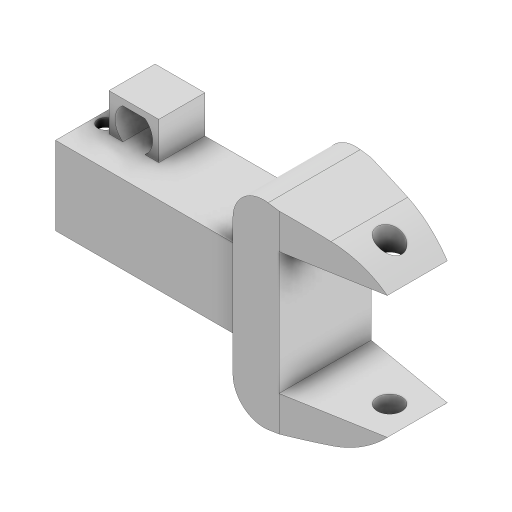
# Autodesk Inventor part: Nuckle
Saved by Autodesk Inventor 2023 (Build 270158000, 158)
## iProperties
Created: 2023-03-23
Part Number: Nuckle
Material: Generic
Document SubType Name: Modeling
Designer: Juyoung Han
Density: 1 g/cm^3
Appearance: Default
Author: Juyoung Han
Autodesk Inventor part; units mm, degrees
ref_plane "YZ Plane" through (0, 0, 0) normal (1, 0, 0) x (0, 1, 0)
ref_plane "XZ Plane" through (0, 0, 0) normal (0, 1, 0) x (-1, 0, 0)
ref_plane "XY Plane" through (0, 0, 0) normal (0, 0, 1) x (1, 0, 0)
sketch "Sketch1" plane through (0, 0, 0) normal (0, 0, 1) x (1, 0, 0)
  line L0 (0, 20) -> (30, 20)
  line L1 (0, 20) -> (0, 0)
  line L2 (-45, 20) -> (-45, 35)
  arc A0 (30, 25) -> (-45, 35) centre (-45, -251.25) ccw
  line L3 (-45, 20) -> (-45, 0)
  line L4 (0, -20) -> (30, -20)
  line L5 (45, -20) -> (45, -20.4834)
  line L6 (0, -20) -> (0, 0)
  line L7 (-45, -20) -> (-45, -35)
  arc A1 (-45, -35) -> (30, -25) centre (-45, 251.25) ccw
  line L8 (-45, -20) -> (-45, 0)
  line L9 (30, 25) -> (30, 20)
  line L10 (30, -25) -> (30, -20)
  point P0 (45, 20.4834)
  point P1 (45, 22.5)
  point P2 (30, 37.5)
  point P3 (-25, -20)
  point P4 (0, -32.987)
  point P5 (45, -22.5)
  point P6 (30, -37.5)
  point P7 (45, -22.5)
  point P8 (30, -37.5)
  dimension "d17" = 15
  constraints: 22 end point, 6 point on circle, 3 point on line, 2 centre point, 2 vertical, 1 horizontal, 1 perpendicular
  measures "d17" distance of L2.start L2.end
extrude "Extrusion1" add sketch "Sketch1" along normal mid plane 30
sketch "Sketch3" plane through (0, -20, 15) normal (0, 1, 0) x (1, 0, 0)
  line L0 (0, 0) -> (0, 30) projected
  line L1 (30, 0) -> (0, 0) projected
  line L2 (0, 30) -> (30, 30) projected
  circle A0 centre (36.5, 15) radius 2
  line L3 (30, 30) -> (30, 0) projected
  point P0 (0, 15)
  dimension "d18" = 4
  constraints: 1 centre point
  measures "d18" diameter of A0
extrude "Extrusion3" cut sketch "Sketch3" along normal through all both and the other way through all contours A0
fillet "Fillet3" radius 30 1 edges at (30, 25, 0)
fillet "Fillet4" radius 30 1 edges at (30, -25, 0)
sketch "Sketch6" plane through (-45, -35, 15) normal (-1, 0, 0) x (0, 0, 1)
  line L0 (-24.0585, 25.4415) -> (-25, 24.5) construction
  line L1 (-4.3571, 37.8214) -> (-10.3571, 37.8214)
  line L2 (-10.3571, 37.8214) -> (-10.3571, 31.8214)
  line L3 (-10.3571, 31.8214) -> (-4.5, 31.8214)
  line L4 (-25, 37.8214) -> (-19, 37.8214)
  line L5 (-19, 37.8214) -> (-19, 31.8214)
  line L6 (-19, 31.8214) -> (-25, 31.8214)
  line L7 (-25, 24.5) -> (-25, 31.8214)
  line L8 (-25, 37.8214) -> (-25, 45)
  line L9 (-4.3571, 45) -> (-4.3571, 37.8214)
  line L10 (-4.5, 31.8214) -> (-4.5, 24.5)
  line L11 (-11.6786, 45) -> (-11.6786, 39)
  line L12 (-11.6786, 39) -> (-17.6786, 39)
  line L13 (-17.6786, 39) -> (-17.6786, 45)
  line L14 (-25, 45) -> (-17.6786, 45)
  line L15 (-11.6786, 45) -> (-4.3571, 45)
  line L16 (-17.6786, 24.5) -> (-17.6786, 30.5)
  line L17 (-17.6786, 30.5) -> (-11.6786, 30.5)
  line L18 (-11.6786, 30.5) -> (-11.6786, 24.5)
  line L19 (-4.5, 24.5) -> (-11.6786, 24.5)
  line L20 (-17.6786, 24.5) -> (-25, 24.5)
  dimension "d59" = 20.5
  dimension "d67" = 6
  dimension "d68" = 6
  dimension "d69" = 6
  dimension "d70" = 6
  dimension "d71" = 6
  dimension "d73" = 6
  constraints: 42 end point, 13 perpendicular, 10 parallel, 3 horizontal
  measures "d59" distance of L10.end L0.end
  measures "d67" distance of L1.end L2.end
  measures "d68" distance of L1.start L1.end
  measures "d69" distance of L4.start L4.end
  measures "d70" distance of L4.end L5.end
  measures "d71" distance of L11.end L12.end
  measures "d73" distance of L16.start L16.end
extrude "Extrusion5" cut sketch "Sketch6" against normal blind 42
sketch "Sketch7" plane through (-45, -35, 15) normal (-1, 0, 0) x (0, 0, 1)
  line L0 (-30, 50) -> (0, 50)
  line L1 (0, 50) -> (0, 20)
  line L2 (0, 20) -> (-30, 20)
  line L3 (-30, 20) -> (-30, 50)
  line L4 (-30, 50) -> (0, 20) construction
  line L5 (0, 50) -> (-30, 20) construction
  line L6 (-22.5355, 32.4645) -> (-22.5355, 28.5251) projected
  line L7 (-24.5355, 32.4645) -> (-22.5355, 32.4645) projected
  line L8 (-24.5355, 25.4645) -> (-24.5355, 32.4645) projected
  line L9 (-17.5355, 25.4645) -> (-24.5355, 25.4645) projected
  line L10 (-17.5355, 27.4645) -> (-17.5355, 25.4645) projected
  line L11 (-21.4749, 27.4645) -> (-17.5355, 27.4645) projected
  line L12 (-17.9393, 31) -> (-21.4749, 27.4645) projected
  line L13 (-12.0607, 31) -> (-17.9393, 31) projected
  line L14 (-8.5251, 27.4645) -> (-12.0607, 31) projected
  line L15 (-12.4645, 27.4645) -> (-8.5251, 27.4645) projected
  line L16 (-12.4645, 25.4645) -> (-12.4645, 27.4645) projected
  line L17 (-5.4645, 25.4645) -> (-12.4645, 25.4645) projected
  line L18 (-5.4645, 32.4645) -> (-5.4645, 25.4645) projected
  line L19 (-7.4645, 32.4645) -> (-5.4645, 32.4645) projected
  line L20 (-7.4645, 28.5251) -> (-7.4645, 32.4645) projected
  line L21 (-11, 32.0607) -> (-7.4645, 28.5251) projected
  line L22 (-11, 37.9393) -> (-11, 32.0607) projected
  line L23 (-7.4645, 41.4749) -> (-11, 37.9393) projected
  line L24 (-7.4645, 37.5355) -> (-7.4645, 41.4749) projected
  line L25 (-5.4645, 37.5355) -> (-7.4645, 37.5355) projected
  line L26 (-5.4645, 44.5355) -> (-5.4645, 37.5355) projected
  line L27 (-12.4645, 44.5355) -> (-5.4645, 44.5355) projected
  line L28 (-12.4645, 42.5355) -> (-12.4645, 44.5355) projected
  line L29 (-8.5251, 42.5355) -> (-12.4645, 42.5355) projected
  line L30 (-12.0607, 39) -> (-8.5251, 42.5355) projected
  line L31 (-17.9393, 39) -> (-12.0607, 39) projected
  line L32 (-21.4749, 42.5355) -> (-17.9393, 39) projected
  line L33 (-17.5355, 42.5355) -> (-21.4749, 42.5355) projected
  line L34 (-17.5355, 44.5355) -> (-17.5355, 42.5355) projected
  line L35 (-24.5355, 44.5355) -> (-17.5355, 44.5355) projected
  line L36 (-24.5355, 37.5355) -> (-24.5355, 44.5355) projected
  line L37 (-22.5355, 37.5355) -> (-24.5355, 37.5355) projected
  line L38 (-22.5355, 41.4749) -> (-22.5355, 37.5355) projected
  line L39 (-19, 37.9393) -> (-22.5355, 41.4749) projected
  line L40 (-19, 32.0607) -> (-19, 37.9393) projected
  line L41 (-22.5355, 28.5251) -> (-19, 32.0607) projected
  line L42 (-30, 70) -> (0, 70) projected
  line L43 (-30, 0) -> (-30, 70) projected
  line L44 (0, 70) -> (0, 0) projected
  line L45 (-30, 0) -> (0, 0) projected
  point P0 (-15, 35)
  dimension "d47" = 30
  dimension "d48" = 30
  constraints: 12 end point, 2 midpoint, 2 parallel, 1 horizontal, 1 perpendicular
  measures "d47" distance of L1.end L2.end
  measures "d48" distance of L0.end L1.end
extrude "Extrusion6" cut sketch "Sketch7" against normal blind 30 contours L43 L42 L44 L0 | L0 L1 L2 L3 | L2 L44 L45 L43 | L6 L41 L40 L39 L38 L37 L36 L35 L34 L33 L32 L31 L30 L29 L28 L27 L26 L25 L24 L23 L22 L21 L20 L19 L18 L17 L16 L15 L14 L13 L12 L11 L10 L9 L8 L7
fillet "Fillet5" radius 10 1 edges at (-15, 33.4236, 0)
fillet "Fillet6" radius 10 1 edges at (-15, -33.4236, 0)
sketch "Sketch8" plane through (0, -20, 15) normal (0, 1, 0) x (1, 0, 0)
  line L0 (0, 0) -> (0, 30) projected
  line L1 (30, 0) -> (0, 0) projected
  line L2 (0, 30) -> (30, 30) projected
  circle A0 centre (36.5, 15) radius 2 projected
  arc A1 (37.9617, 6.6266) -> (37.9617, 23.3734) centre (36.5, 15) ccw
  line L3 (0, 0) -> (37.9617, 6.6266)
  line L4 (0, 30) -> (37.9617, 23.3734)
  line L5 (-15, 0) -> (-15, 30) projected
  line L6 (0, 0) -> (-15, 0)
  line L7 (-15, 0) -> (-15, 30)
  line L8 (-15, 0) -> (-15, 30)
  line L9 (0, 12.4645) -> (0, 5.4645) projected
  line L10 (-15, 30) -> (0, 30)
  line L11 (-3.552, 30) -> (-3.552, 0) projected
  line L12 (30, 30) -> (30, 0) projected
  point P0 (0, 15)
  constraints: 12 end point, 2 perpendicular, 2 point on circle, 2 tangent, 1 centre point, 1 coincident, 1 parallel
extrude "Extrusion7" cut sketch "Sketch8" along normal through all both and the other way through all contours L6 L11 L10 L0 | L0 L4 L12 L3 | L12 L4 A1 L3 | L6 L5 L10 L11 | A0 keep common part
sketch "Sketch9" plane through (0, -20, 15) normal (0, 1, 0) x (1, 0, 0)
  circle A0 centre (21, 15) radius 4
  line L0 (30, 24.7632) -> (30, 5.2368) projected
  point P0 (0, 15)
  point P1 (30, 15)
  dimension "d55" = 8
  dimension "d56" = 9
  constraints: 1 centre point, 1 midpoint
  measures "d55" diameter of A0
  measures "d56" distance of point (30, 15) A0.centre
extrude "Extrusion8" cut sketch "Sketch9" along normal through all both and the other way through all
sketch "Sketch10" plane through (-15, -35, 15) normal (-1, 0, 0) x (0, 0, 1)
  point P0 (-15, 35)
sketch "Sketch11" plane through (-15, -35, 15) normal (-1, 0, 0) x (0, 0, 1)
  line L0 (-25, 45) -> (-17.6786, 45) projected
  line L1 (-4.5, 24.5) -> (-11.6786, 24.5) projected
  line L2 (-27.75, 22.25) -> (-2.25, 22.25)
  line L3 (-2.25, 22.25) -> (-2.25, 47.75)
  line L4 (-2.25, 47.75) -> (-27.75, 47.75)
  line L5 (-27.75, 47.75) -> (-27.75, 22.25)
  line L6 (-17.6786, 45) -> (-17.6786, 39) projected
  line L7 (-17.6786, 45) -> (-17.6786, 39)
  line L8 (-17.6786, 39) -> (-11.6786, 39) projected
  line L9 (-17.6786, 39) -> (-11.6786, 39)
  line L10 (-11.6786, 39) -> (-11.6786, 45) projected
  line L11 (-11.6786, 39) -> (-11.6786, 45)
  line L12 (-10.3571, 37.8214) -> (-4.3571, 37.8214) projected
  line L13 (-4.3571, 37.8214) -> (-10.3571, 37.8214)
  line L14 (-10.3571, 37.8214) -> (-10.3571, 31.8214) projected
  line L15 (-10.3571, 37.8214) -> (-10.3571, 31.8214)
  line L16 (-4.5, 31.8214) -> (-10.3571, 31.8214) projected
  line L17 (-10.3571, 31.8214) -> (-4.5, 31.8214)
  line L18 (-11.6786, 30.5) -> (-11.6786, 24.5) projected
  line L19 (-11.6786, 24.5) -> (-11.6786, 30.5)
  line L20 (-17.6786, 30.5) -> (-11.6786, 30.5) projected
  line L21 (-11.6786, 30.5) -> (-17.6786, 30.5)
  line L22 (-17.6786, 30.5) -> (-17.6786, 24.5) projected
  line L23 (-17.6786, 30.5) -> (-17.6786, 24.5)
  line L24 (-19, 37.8214) -> (-25, 37.8214) projected
  line L25 (-25, 37.8214) -> (-19, 37.8214)
  line L26 (-25, 31.8214) -> (-19, 31.8214) projected
  line L27 (-19, 37.8214) -> (-19, 31.8214)
  line L28 (-19, 31.8214) -> (-25, 31.8214)
  line L29 (-25, 45) -> (-17.6786, 45)
  line L30 (-11.6786, 45) -> (-4.5, 45)
  line L31 (-25, 24.5) -> (-25, 31.8214)
  line L32 (-25, 37.8214) -> (-25, 45)
  line L33 (-4.5, 24.5) -> (-11.6786, 24.5)
  line L34 (-17.6786, 24.5) -> (-25, 24.5)
  line L35 (-4.5, 45) -> (-4.5, 37.8214)
  line L36 (-4.5, 31.8214) -> (-4.5, 24.5)
  point P0 (-15, 35)
  constraints: 48 end point, 10 parallel, 10 perpendicular, 7 collinear, 4 horizontal, 1 point on line
extrude "Extrusion9" add sketch "Sketch11" along normal blind 45
sketch "Sketch12" plane through (-60, -35, 15) normal (-1, 0, 0) x (0, 0, 1)
  line L0 (-17.6786, 45) -> (-17.6786, 39) projected
  line L1 (-17.6786, 45) -> (-17.6786, 39)
  line L2 (-17.6786, 39) -> (-11.6786, 39) projected
  line L3 (-17.6786, 39) -> (-11.6786, 39)
  line L4 (-11.6786, 39) -> (-11.6786, 45) projected
  line L5 (-11.6786, 39) -> (-11.6786, 45)
  line L6 (-11.6786, 45) -> (-17.6786, 45)
  line L7 (-11.6786, 30.5) -> (-17.6786, 30.5) projected
  line L8 (-17.6786, 30.5) -> (-11.6786, 30.5)
  line L9 (-11.6786, 24.5) -> (-11.6786, 30.5) projected
  line L10 (-11.6786, 30.5) -> (-11.6786, 24.5)
  line L11 (-17.6786, 24.5) -> (-25, 24.5) projected
  line L12 (-11.6786, 24.5) -> (-17.6786, 24.5)
  line L13 (-17.6786, 24.5) -> (-17.6786, 30.5)
  point P0 (-15, 35)
  constraints: 16 end point, 5 collinear, 2 perpendicular, 1 horizontal
extrude "Extrusion10" cut sketch "Sketch12" against normal up to surface (57 mm away)
sketch "Sketch13" plane through (-15, 12.75, 12.75) normal (0, 1, 0) x (1, 0, 0)
  point P0 (15, 12.75)
sketch "Sketch15" plane through (-15, -12.75, -12.75) normal (0, 0, -1) x (-1, 0, 0)
  line L0 (0, 25.5) -> (45, 25.5) projected
  line L1 (41.4, 35.7) -> (45, 35.7)
  arc A0 (41.4, 35.7) -> (41.4, 25.5) centre (45.352, 30.6) ccw
  line L2 (48.6, 35.7) -> (45, 35.7)
  arc A1 (48.6, 25.5) -> (48.6, 35.7) centre (44.648, 30.6) ccw
  line L3 (0, 25.5) -> (45, 25.5) projected
  line L4 (0, 22.75) -> (45, 22.75) projected
  line L5 (45, 37.7) -> (36.9, 37.7)
  line L6 (36.9, 37.7) -> (36.9, 25.5)
  line L7 (45, 37.7) -> (53.1, 37.7)
  line L8 (53.1, 37.7) -> (53.1, 25.5)
  line L9 (36.9, 25.5) -> (41.4, 25.5)
  line L10 (48.6, 25.5) -> (53.1, 25.5)
  line L11 (45, 0) -> (45, 25.5) projected
  point P0 (-15, 12.75)
  point P1 (38.9, 25.5)
  point P2 (38.9, 35.7)
  point P3 (51.1, 25.5)
  point P4 (51.1, 35.7)
  dimension "d85" = 10.2
  constraints: 16 end point, 4 point on circle, 2 centre point, 2 perpendicular, 2 point on line, 1 collinear
  measures "d85" distance of point (38.9, 25.5) point (38.9, 35.7)
extrude "Extrusion12" add sketch "Sketch15" against normal blind 15
sketch "Sketch16" plane through (-60, -35, 15) normal (-1, 0, 0) x (0, 0, 1)
  line L0 (-4.5, 24.5) -> (-25, 24.5) projected
  line L1 (-25, 24.5) -> (-25, 31.8214) projected
  line L2 (-25, 31.8214) -> (-19, 31.8214) projected
  line L3 (-19, 31.8214) -> (-19, 37.8214) projected
  line L4 (-19, 37.8214) -> (-25, 37.8214) projected
  line L5 (-25, 37.8214) -> (-25, 45) projected
  line L6 (-25, 45) -> (-4.5, 45) projected
  line L7 (-4.5, 45) -> (-4.5, 37.8214) projected
  line L8 (-4.5, 37.8214) -> (-10.3571, 37.8214) projected
  line L9 (-10.3571, 37.8214) -> (-10.3571, 31.8214) projected
  line L10 (-10.3571, 31.8214) -> (-4.5, 31.8214) projected
  line L11 (-4.5, 31.8214) -> (-4.5, 24.5) projected
  line L12 (-2.25, 22.25) -> (-2.25, 47.75) projected
  line L13 (-2.25, 47.75) -> (-27.75, 47.75) projected
  line L14 (-27.75, 47.75) -> (-27.75, 22.25) projected
  line L15 (-27.75, 22.25) -> (-2.25, 22.25) projected
  point P0 (-15, 35)
extrude "Extrusion13" add sketch "Sketch16" along normal blind 15
sketch "Sketch17" plane through (-15, 12.75, 12.75) normal (0, 1, 0) x (1, 0, 0)
  circle A0 centre (-56.5, 12.75) radius 2.5
  line L0 (-60, 0) -> (-60, 25.5) projected
  point P0 (15, 12.75)
  dimension "d96" = 5
  dimension "d97" = 3.5
  constraints: 1 centre point
  measures "d96" diameter of A0
  measures "d97" distance from line of L0 A0.centre
extrude "Extrusion14" cut sketch "Sketch17" against normal through all
body "Solid1"
